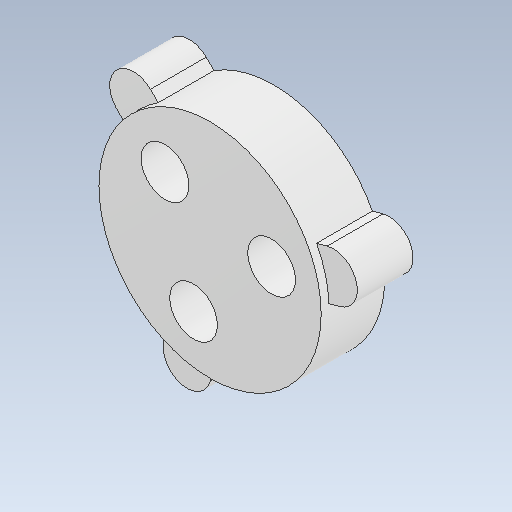
# Autodesk Inventor part: アームカムFD18t4
Saved by Autodesk Inventor 2020.2 (Build 242310000, 310)
## iProperties
Created: 2020-03-20
Part Number: アームカムFD18t4
Material: アセタール樹脂、白
Document SubType Name: Modeling
Designer: aoyam
Density: 1.425 g/cm^3
Appearance: 滑らか - 白
Mass: 1.25719 g
Surface Area: 7.99457 cm^2
Volume: 0.882239 cm^3
Author: aoyam
Autodesk Inventor part; units mm, degrees
ref_plane "YZ Plane" through (0, 0, 0) normal (1, 0, 0) x (0, 1, 0)
ref_plane "XZ Plane" through (0, 0, 0) normal (0, 1, 0) x (-1, 0, 0)
ref_plane "XY Plane" through (0, 0, 0) normal (0, 0, 1) x (1, 0, 0)
sketch "スケッチ1" plane through (0, 0, 0) normal (0, 0, 1) x (1, 0, 0)
  circle A0 centre (0, 0) radius 6.975
  circle A1 centre (-2.8284, 2.8284) radius 1.5
  circle A2 centre (-1.0353, -3.8637) radius 1.5
  circle A3 centre (3.8637, 1.0353) radius 1.5
  circle A4 centre (0, 0) radius 9
  line L0 (0, 0) -> (7.2444, 1.9411) construction
  line L1 (0.3882, -1.4489) -> (7.6327, 0.4923)
  line L2 (6.8562, 3.39) -> (-0.3882, 1.4489)
  arc A5 (-0.3882, 1.4489) -> (0.3882, -1.4489) centre (0, 0) ccw
  arc A6 (7.6327, 0.4923) -> (6.8562, 3.39) centre (7.2444, 1.9411) ccw
  arc A7 (-4.2426, 6.364) -> (-6.364, 4.2426) centre (-5.3033, 5.3033) ccw
  line L3 (1.0607, 1.0607) -> (-4.2426, 6.364)
  line L4 (-6.364, 4.2426) -> (-1.0607, -1.0607)
  arc A8 (-3.39, -6.8562) -> (-0.4923, -7.6327) centre (-1.9411, -7.2444) ccw
  line L5 (-1.4489, 0.3882) -> (-3.39, -6.8562)
  line L6 (-0.4923, -7.6327) -> (1.4489, -0.3882)
  point P0 (3.6222, 0.9706)
  point P1 (6.1915, 3.2119)
  point P2 (6.9679, 0.3141)
  point P3 (-5.8773, 3.756)
  point P4 (-3.756, 5.8773)
  point P5 (-0.3141, -6.9679)
  point P6 (-3.2119, -6.1915)
  dimension "d0" = 13.95
  dimension "d1" = 3
  dimension "d2" = 4
  dimension "d5" = 360
  dimension "d9" = 18
  dimension "d14" = 3
  dimension "d17" = 360
  constraints: 16 end point, 9 centre point, 8 point on circle, 5 tangent, 2 coincident, 1 midpoint, 1 parallel, 1 point on line, 32 other
  measures "d0" diameter of A0
  measures "d1" diameter of A1
  measures "d2" distance of A1.centre point (0, 0)
  measures "d9" diameter of A4
  measures "d14" diameter of A6
extrude "押し出し2" add sketch "スケッチ1" along normal blind 4 contours A0 L6 L1 | L1 A3 L2 A0 | A0 L5 A2 L6 | L2 L3 A0 | L1 A5 L2 A3 | A0 L4 L5 | A2 L5 L4 A5 L1 L6 | L3 A1 L4 A0 | L3 L2 A5 L5 L4 A1 | L5 A5 L4
extrude "押し出し3" add sketch "スケッチ1" along normal blind 3.5 contours A0 L2 A6 L1 | L6 A8 L5 A0 | A0 L4 A7 L3
